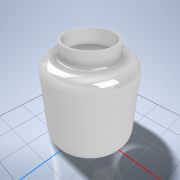
# Autodesk Inventor part: garnek
Saved by Autodesk Inventor 2021 (Build 250183000, 183)
## iProperties
Created: 2021-05-20
Part Number: garnek
Material: Stal nierdzewna, szczotkowana
Document SubType Name: Modeling
Designer: Wojciech Wołczek
Density: 8 g/cm^3
Appearance: Obrobione — aluminium
Author: Wojciech Wołczek
Autodesk Inventor part; units mm, degrees
ref_plane "YZ Plane" through (0, 0, 0) normal (1, 0, 0) x (0, 1, 0)
ref_plane "XZ Plane" through (0, 0, 0) normal (0, 1, 0) x (-1, 0, 0)
ref_plane "XY Plane" through (0, 0, 0) normal (0, 0, 1) x (1, 0, 0)
sketch "Szkic1" plane through (0, 0, 0) normal (0, 0, 1) x (1, 0, 0)
  line L0 (0, 0) -> (110, 0)
  line L1 (150, 40) -> (150, 260)
  line L2 (150, 350) -> (0, 350)
  line L3 (0, 350) -> (0, 0)
  arc A0 (110, 0) -> (150, 40) centre (110, 40) ccw
  line L4 (0, 350) -> (90, 350)
  line L5 (90, 350) -> (90, 310)
  line L6 (0, 300) -> (0, 350)
  line L7 (100, 300) -> (110, 300)
  arc A1 (150, 260) -> (110, 300) centre (110, 260) ccw
  arc A2 (90, 310) -> (100, 300) centre (100, 310) ccw
  line L8 (80, 310) -> (80, 340)
  line L9 (80, 340) -> (10, 340)
  line L10 (10, 340) -> (10, 10)
  line L11 (10, 10) -> (110, 10)
  arc A3 (110, 10) -> (140, 40) centre (110, 40) ccw
  line L12 (140, 40) -> (140, 260)
  arc A4 (140, 260) -> (110, 290) centre (110, 260) ccw
  line L13 (110, 290) -> (100, 290)
  arc A5 (80, 310) -> (100, 290) centre (100, 310) ccw
  line L14 (80, 340) -> (80, 350)
  line L15 (10, 10) -> (0, 10)
  point P0 (150, 0)
  point P1 (90, 300)
  point P2 (150, 300)
  dimension "d0" = 150
  dimension "d1" = 350
  dimension "d2" = 40
  dimension "d3" = 90
  dimension "d4" = 50
  dimension "d5" = 40
  dimension "d6" = 10
  dimension "d7" = 10
  constraints: 32 end point, 12 point on circle, 9 point on line, 6 centre point, 6 tangent, 5 perpendicular, 4 parallel, 2 horizontal, 1 vertical, 8 other
  measures "d0" distance of L2.end L2.start
  measures "d1" distance of L2.start point (150, 0)
  measures "d2" radius of A0
  measures "d3" distance of point (90, 300) L6.start
  measures "d4" distance of L4.end point (90, 300)
  measures "d5" radius of A1
  measures "d6" radius of A2
  measures "d7" distance between parallel lines of L5 L8
revolve "Obrót1" add sketch "Szkic1" angle 360 about axis through (0, 350, 0) along (0, -1, 0) contours L3 L15 L11 A3 L12 A4 L13 A5 L8 L14 L2 L5 A2 L7 A1 L1 A0 L0
